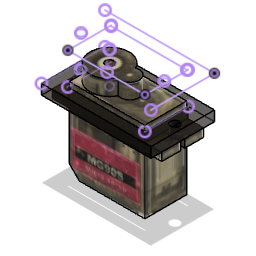
Servo v2 (Autodesk Fusion 360 design; units mm, degrees)
Autodesk Fusion 360 part; units mm, degrees
(part 1 of 2)
sketch "Component_Variables" plane through (0, 0, 0) normal (0, 1, 0) x (1, 0, 0) in component "Servo"
  dimension "tol" = 0
  dimension "tol2" = 0
  dimension "HornScrewtopThickness" = 1.2
  dimension "HornCollarGap" = 0.35
  dimension "HornToServoTopGap" = 0.2
  dimension "HornScrewtopScrewDiaExtra" = 0.4
sketch "Shaft" plane through (0, 0, 0) normal (0, 1, 0) x (1, 0, 0) in component "Shaft"
  circle A0 centre (0, 0) radius 1.25
  circle A1 centre (0, 0) radius 2.4
  circle A2 centre (0, 0) radius 2.25 construction
  line L0 (0, 0) -> (0, 2.4) construction
  line L1 (0, 0) -> (-0.741641, 2.282536) construction
  line L2 (-0.695288, 2.139877) -> (0, 2.25) construction
  line L3 (-0.347644, 2.194939) -> (-0.375443, 2.370452) construction
  line L4 (0, 2.4) -> (-4, 2.4) construction
  line L5 (-0.351978, 2.222299) -> (-1.537204, 2.034577) construction
  spline S0 degree 5 poles (0, 2.4) (-0.019472, 2.4) (-0.055772, 2.396788) (-0.102302, 2.382342) (-0.151568, 2.347419) (-0.205208, 2.293022) (-0.253386, 2.253987) (-0.298375, 2.233713) (-0.333289, 2.225259) (-0.351978, 2.222299) knots 0 0 0 0 0 0 0.2 0.4 0.6 0.8 1 1 1 1 1 1
  line L6 (0.047124, 2.4) -> (-0.047124, 2.4)
  line L7 (-0.305434, 2.229671) -> (-0.398521, 2.214927)
  spline S1 degree 5 poles (0, 2.4) (0.019472, 2.4) (0.055772, 2.396788) (0.102302, 2.382342) (0.151568, 2.347419) (0.205208, 2.293022) (0.253386, 2.253987) (0.298375, 2.233713) (0.333289, 2.225259) (0.351978, 2.222299) knots 0 0 0 0 0 0 0.2 0.4 0.6 0.8 1 1 1 1 1 1
  line L8 (-0.047124, 2.4) -> (0.047124, 2.4)
  line L9 (0.305434, 2.229671) -> (0.398521, 2.214927)
  line L10 (0.351978, 2.222299) -> (0, 0)
  line L11 (-0.351978, 2.222299) -> (0, 0)
  circle A3 centre (0, 0) radius 1.75
  spline S2 degree 5 poles (-0.741641, 2.282536) (-0.723122, 2.288553) (-0.687606, 2.296715) (-0.638889, 2.297355) (-0.581243, 2.279365) (-0.513418, 2.244207) (-0.455536, 2.22197) (-0.406484, 2.21659) (-0.370666, 2.219339) (-0.351978, 2.222299) knots 0 0 0 0 0 0 0.2 0.4 0.6 0.8 1 1 1 1 1 1
  line L12 (-0.786458, 2.267974) -> (-0.696823, 2.297098)
  line L13 (-0.398521, 2.214927) -> (-0.305434, 2.229671)
  point P0 (-0.741641, 2.282536)
  point P1 (-1.410685, 1.941641)
  point P2 (-1.941641, 1.410685)
  point P3 (-2.282536, 0.741641)
  point P4 (-0.347644, 2.194939)
  point P5 (-2.4, 0)
  point P6 (-2.282536, -0.741641)
  point P7 (-1.941641, -1.410685)
  point P8 (-1.410685, -1.941641)
  point P9 (-0.741641, -2.282536)
  point P10 (0, -2.4)
  point P11 (0.741641, -2.282536)
  point P12 (1.410685, -1.941641)
  point P13 (1.941641, -1.410685)
  point P14 (2.282536, -0.741641)
  point P15 (2.4, 0)
  point P16 (2.282536, 0.741641)
  point P17 (1.941641, 1.410685)
  point P18 (1.410685, 1.941641)
  point P19 (0.741641, 2.282536)
  dimension "ScrewholeDia" = 2.5
  dimension "ShaftOuterDia" = 4.8
  dimension "ShaftSplinesInnerDia" = 4.5
  dimension "d5" = 360
  dimension "d6" = 4
  dimension "d7" = 1.2
  dimension "SplineTipPointiness" = 0.094248
  dimension "SplineInnerPointiness" = 0.094248
  dimension "d13" = 3.5
  constraint coincident A0.centre A1.centre
  constraint concentric A0 A1
  constraint concentric A0 A2
  constraint coincident A1 L0.end
  constraint vertical L0
  constraint coincident A2 L2.end
  constraint coincident L0 L2.end
  constraint perpendicular L2 L3
  constraint tangent A1 L4
  constraint perpendicular L3 L5
  constraint midpoint L0.end L6
  constraint parallel L4 L6
  constraint parallel L5 L7
  constraint symmetric L4.start L0 S0.start
  constraint concentric A1 A3
  measures "ScrewholeDia" diameter of A0
  measures "ShaftOuterDia" diameter of A1
  measures "ShaftSplinesInnerDia" diameter of A2
  measures "d6" distance of L0.end L4.end
  measures "d13" diameter of A3
extrude "Extrude3" add sketch "Shaft" against normal blind 3.5 contours A0 L10 L11 | A0 L10 L11 A3 | A0 L10 L11 | A0 L10 L11 A3 | S0 S1 L10 L11 A3 | A1 S1 L10 L11 A3 S2 | A1 S0 S2 picked at (0.828843, -0.061007) picked at (1.484688, -0.538585) picked at (-0.086988, 0.827632) picked at (0.143589, 1.574781) picked at (0.030529, 2.097713) picked at (-0.857161, 2.002429) picked at (-0.367278, 2.318902) makes body 1 in component "Shaft"
extrude "Extrude4" cut sketch "Shaft" against normal blind 3.5 contours A0 L10 L11 | A0 L10 L11 | A1 S0 S2 picked at (0.828843, -0.061007) picked at (-0.086988, 0.827632) picked at (-0.367278, 2.318902) bodies 1 in component "Shaft"
pattern_circular "C-Pattern3" count 20 over 360 about axis through (0, 1.75, 0) along (0, 1, 0) of "Extrude4" in component "Shaft"
extrude "Ignore" add sketch "Shaft" along normal blind 3.5 separate body contours A0 L10 L11 A3 | S0 S1 L10 L11 A3 picked at (-0.186964, 1.570222) picked at (-0.030529, 2.097713) makes body 2 in component "Shaft"
coil "CoilPrimitive1" add diameter 2.5 section triangle in size 0.2 inside turns 8.75 pitch 0.4 right hand placed x (1, 0, 0) y (0, 0, 1) z (0, -1, 0) at (0, 0, 0) separate body makes body 3 in component "Shaft"
extrude "Extrude5" add sketch "Shaft" against normal blind 3.5 separate body contours A0 L10 L11 | A0 L10 L11 picked at (0.828843, -0.061007) picked at (0.086988, 0.827632) makes body 4 in component "Shaft"
combine "Combine2" operation intersect target body 4 tool bodies 3 in component "Shaft"
sketch "Hat" plane through (0, -3.5, 0) normal (0, -1, 0) x (1, 0, 0) in component "Servo"
  circle A0 centre (0, 0) radius 1.25
  spline S0 degree 5 poles (0, -2.4) (0.019472, -2.4) (0.055772, -2.396788) (0.102302, -2.382342) (0.151568, -2.347419) (0.205208, -2.293022) (0.253386, -2.253987) (0.298375, -2.233713) (0.333289, -2.225259) (0.351978, -2.222299) knots 0 0 0 0 0 0 0.2 0.4 0.6 0.8 1 1 1 1 1 1
  spline S1 degree 5 poles (0.351978, -2.222299) (0.370666, -2.219339) (0.406484, -2.21659) (0.455536, -2.22197) (0.513418, -2.244207) (0.581243, -2.279365) (0.638889, -2.297355) (0.687606, -2.296715) (0.723122, -2.288553) (0.741641, -2.282536) knots -1 -1 -1 -1 -1 -1 -0.8 -0.6 -0.4 -0.2 0 0 0 0 0 0
  spline S2 degree 5 poles (0.741641, -2.282536) (0.760159, -2.276519) (0.79369, -2.262246) (0.833479, -2.234128) (0.869542, -2.185691) (0.903747, -2.117381) (0.937505, -2.065369) (0.974026, -2.032184) (1.004619, -2.013355) (1.021479, -2.004765) knots 0 0 0 0 0 0 0.2 0.4 0.6 0.8 1 1 1 1 1 1
  spline S3 degree 5 poles (1.021479, -2.004765) (1.038338, -1.996174) (1.071553, -1.982492) (1.119867, -1.972451) (1.181788, -1.975712) (1.257157, -1.988191) (1.317541, -1.987487) (1.363676, -1.971824) (1.394932, -1.953086) (1.410685, -1.941641) knots -1 -1 -1 -1 -1 -1 -0.8 -0.6 -0.4 -0.2 0 0 0 0 0 0
  spline S4 degree 5 poles (1.410685, -1.941641) (1.426437, -1.930196) (1.453917, -1.90626) (1.483069, -1.867223) (1.502399, -1.810012) (1.513821, -1.734476) (1.529854, -1.674577) (1.554334, -1.631731) (1.577611, -1.60437) (1.59099, -1.59099) knots 0 0 0 0 0 0 0.2 0.4 0.6 0.8 1 1 1 1 1 1
  spline S5 degree 5 poles (1.59099, -1.59099) (1.60437, -1.577611) (1.631731, -1.554334) (1.674577, -1.529854) (1.734476, -1.513821) (1.810012, -1.502399) (1.867223, -1.483069) (1.90626, -1.453917) (1.930196, -1.426437) (1.941641, -1.410685) knots -1 -1 -1 -1 -1 -1 -0.8 -0.6 -0.4 -0.2 0 0 0 0 0 0
  spline S6 degree 5 poles (1.941641, -1.410685) (1.953086, -1.394932) (1.971824, -1.363676) (1.987487, -1.317541) (1.988191, -1.257157) (1.975712, -1.181788) (1.972451, -1.119867) (1.982492, -1.071553) (1.996174, -1.038338) (2.004765, -1.021479) knots 0 0 0 0 0 0 0.2 0.4 0.6 0.8 1 1 1 1 1 1
  spline S7 degree 5 poles (2.004765, -1.021479) (2.013355, -1.004619) (2.032184, -0.974026) (2.065369, -0.937505) (2.117381, -0.903747) (2.185691, -0.869542) (2.234128, -0.833479) (2.262246, -0.79369) (2.276519, -0.760159) (2.282536, -0.741641) knots -1 -1 -1 -1 -1 -1 -0.8 -0.6 -0.4 -0.2 0 0 0 0 0 0
  spline S8 degree 5 poles (2.282536, -0.741641) (2.288553, -0.723122) (2.296715, -0.687606) (2.297355, -0.638889) (2.279365, -0.581243) (2.244207, -0.513418) (2.22197, -0.455536) (2.21659, -0.406484) (2.219339, -0.370666) (2.222299, -0.351978) knots 0 0 0 0 0 0 0.2 0.4 0.6 0.8 1 1 1 1 1 1
  spline S9 degree 5 poles (2.222299, -0.351978) (2.225259, -0.333289) (2.233713, -0.298375) (2.253987, -0.253386) (2.293022, -0.205208) (2.347419, -0.151568) (2.382342, -0.102302) (2.396788, -0.055772) (2.4, -0.019472) (2.4, 0) knots -1 -1 -1 -1 -1 -1 -0.8 -0.6 -0.4 -0.2 0 0 0 0 0 0
  spline S10 degree 5 poles (2.4, 0) (2.4, 0.019472) (2.396788, 0.055772) (2.382342, 0.102302) (2.347419, 0.151568) (2.293022, 0.205208) (2.253987, 0.253386) (2.233713, 0.298375) (2.225259, 0.333289) (2.222299, 0.351978) knots 0 0 0 0 0 0 0.2 0.4 0.6 0.8 1 1 1 1 1 1
  spline S11 degree 5 poles (2.222299, 0.351978) (2.219339, 0.370666) (2.21659, 0.406484) (2.22197, 0.455536) (2.244207, 0.513418) (2.279365, 0.581243) (2.297355, 0.638889) (2.296715, 0.687606) (2.288553, 0.723122) (2.282536, 0.741641) knots -1 -1 -1 -1 -1 -1 -0.8 -0.6 -0.4 -0.2 0 0 0 0 0 0
  spline S12 degree 5 poles (2.282536, 0.741641) (2.276519, 0.760159) (2.262246, 0.79369) (2.234128, 0.833479) (2.185691, 0.869542) (2.117381, 0.903747) (2.065369, 0.937505) (2.032184, 0.974026) (2.013355, 1.004619) (2.004765, 1.021479) knots 0 0 0 0 0 0 0.2 0.4 0.6 0.8 1 1 1 1 1 1
  spline S13 degree 5 poles (2.004765, 1.021479) (1.996174, 1.038338) (1.982492, 1.071553) (1.972451, 1.119867) (1.975712, 1.181788) (1.988191, 1.257157) (1.987487, 1.317541) (1.971824, 1.363676) (1.953086, 1.394932) (1.941641, 1.410685) knots -1 -1 -1 -1 -1 -1 -0.8 -0.6 -0.4 -0.2 0 0 0 0 0 0
  spline S14 degree 5 poles (1.941641, 1.410685) (1.930196, 1.426437) (1.90626, 1.453917) (1.867223, 1.483069) (1.810012, 1.502399) (1.734476, 1.513821) (1.674577, 1.529854) (1.631731, 1.554334) (1.60437, 1.577611) (1.59099, 1.59099) knots 0 0 0 0 0 0 0.2 0.4 0.6 0.8 1 1 1 1 1 1
  spline S15 degree 5 poles (1.59099, 1.59099) (1.577611, 1.60437) (1.554334, 1.631731) (1.529854, 1.674577) (1.513821, 1.734476) (1.502399, 1.810012) (1.483069, 1.867223) (1.453917, 1.90626) (1.426437, 1.930196) (1.410685, 1.941641) knots -1 -1 -1 -1 -1 -1 -0.8 -0.6 -0.4 -0.2 0 0 0 0 0 0
  spline S16 degree 5 poles (1.410685, 1.941641) (1.394932, 1.953086) (1.363676, 1.971824) (1.317541, 1.987487) (1.257157, 1.988191) (1.181788, 1.975712) (1.119867, 1.972451) (1.071553, 1.982492) (1.038338, 1.996174) (1.021479, 2.004765) knots 0 0 0 0 0 0 0.2 0.4 0.6 0.8 1 1 1 1 1 1
  spline S17 degree 5 poles (1.021479, 2.004765) (1.004619, 2.013355) (0.974026, 2.032184) (0.937505, 2.065369) (0.903747, 2.117381) (0.869542, 2.185691) (0.833479, 2.234128) (0.79369, 2.262246) (0.760159, 2.276519) (0.741641, 2.282536) knots -1 -1 -1 -1 -1 -1 -0.8 -0.6 -0.4 -0.2 0 0 0 0 0 0
  spline S18 degree 5 poles (0.741641, 2.282536) (0.723122, 2.288553) (0.687606, 2.296715) (0.638889, 2.297355) (0.581243, 2.279365) (0.513418, 2.244207) (0.455536, 2.22197) (0.406484, 2.21659) (0.370666, 2.219339) (0.351978, 2.222299) knots 0 0 0 0 0 0 0.2 0.4 0.6 0.8 1 1 1 1 1 1
  spline S19 degree 5 poles (0.351978, 2.222299) (0.333289, 2.225259) (0.298375, 2.233713) (0.253386, 2.253987) (0.205208, 2.293022) (0.151568, 2.347419) (0.102302, 2.382342) (0.055772, 2.396788) (0.019472, 2.4) (0, 2.4) knots -1 -1 -1 -1 -1 -1 -0.8 -0.6 -0.4 -0.2 0 0 0 0 0 0
  spline S20 degree 5 poles (0, 2.4) (-0.019472, 2.4) (-0.055772, 2.396788) (-0.102302, 2.382342) (-0.151568, 2.347419) (-0.205208, 2.293022) (-0.253386, 2.253987) (-0.298375, 2.233713) (-0.333289, 2.225259) (-0.351978, 2.222299) knots 0 0 0 0 0 0 0.2 0.4 0.6 0.8 1 1 1 1 1 1
  spline S21 degree 5 poles (-0.351978, 2.222299) (-0.370666, 2.219339) (-0.406484, 2.21659) (-0.455536, 2.22197) (-0.513418, 2.244207) (-0.581243, 2.279365) (-0.638889, 2.297355) (-0.687606, 2.296715) (-0.723122, 2.288553) (-0.741641, 2.282536) knots -1 -1 -1 -1 -1 -1 -0.8 -0.6 -0.4 -0.2 0 0 0 0 0 0
  spline S22 degree 5 poles (-0.741641, 2.282536) (-0.760159, 2.276519) (-0.79369, 2.262246) (-0.833479, 2.234128) (-0.869542, 2.185691) (-0.903747, 2.117381) (-0.937505, 2.065369) (-0.974026, 2.032184) (-1.004619, 2.013355) (-1.021479, 2.004765) knots 0 0 0 0 0 0 0.2 0.4 0.6 0.8 1 1 1 1 1 1
  spline S23 degree 5 poles (-1.021479, 2.004765) (-1.038338, 1.996174) (-1.071553, 1.982492) (-1.119867, 1.972451) (-1.181788, 1.975712) (-1.257157, 1.988191) (-1.317541, 1.987487) (-1.363676, 1.971824) (-1.394932, 1.953086) (-1.410685, 1.941641) knots -1 -1 -1 -1 -1 -1 -0.8 -0.6 -0.4 -0.2 0 0 0 0 0 0
  spline S24 degree 5 poles (-1.410685, 1.941641) (-1.426437, 1.930196) (-1.453917, 1.90626) (-1.483069, 1.867223) (-1.502399, 1.810012) (-1.513821, 1.734476) (-1.529854, 1.674577) (-1.554334, 1.631731) (-1.577611, 1.60437) (-1.59099, 1.59099) knots 0 0 0 0 0 0 0.2 0.4 0.6 0.8 1 1 1 1 1 1
  spline S25 degree 5 poles (-1.59099, 1.59099) (-1.60437, 1.577611) (-1.631731, 1.554334) (-1.674577, 1.529854) (-1.734476, 1.513821) (-1.810012, 1.502399) (-1.867223, 1.483069) (-1.90626, 1.453917) (-1.930196, 1.426437) (-1.941641, 1.410685) knots -1 -1 -1 -1 -1 -1 -0.8 -0.6 -0.4 -0.2 0 0 0 0 0 0
  spline S26 degree 5 poles (-1.941641, 1.410685) (-1.953086, 1.394932) (-1.971824, 1.363676) (-1.987487, 1.317541) (-1.988191, 1.257157) (-1.975712, 1.181788) (-1.972451, 1.119867) (-1.982492, 1.071553) (-1.996174, 1.038338) (-2.004765, 1.021479) knots 0 0 0 0 0 0 0.2 0.4 0.6 0.8 1 1 1 1 1 1
  spline S27 degree 5 poles (-2.004765, 1.021479) (-2.013355, 1.004619) (-2.032184, 0.974026) (-2.065369, 0.937505) (-2.117381, 0.903747) (-2.185691, 0.869542) (-2.234128, 0.833479) (-2.262246, 0.79369) (-2.276519, 0.760159) (-2.282536, 0.741641) knots -1 -1 -1 -1 -1 -1 -0.8 -0.6 -0.4 -0.2 0 0 0 0 0 0
  spline S28 degree 5 poles (-2.282536, 0.741641) (-2.288553, 0.723122) (-2.296715, 0.687606) (-2.297355, 0.638889) (-2.279365, 0.581243) (-2.244207, 0.513418) (-2.22197, 0.455536) (-2.21659, 0.406484) (-2.219339, 0.370666) (-2.222299, 0.351978) knots 0 0 0 0 0 0 0.2 0.4 0.6 0.8 1 1 1 1 1 1
  spline S29 degree 5 poles (-2.222299, 0.351978) (-2.225259, 0.333289) (-2.233713, 0.298375) (-2.253987, 0.253386) (-2.293022, 0.205208) (-2.347419, 0.151568) (-2.382342, 0.102302) (-2.396788, 0.055772) (-2.4, 0.019472) (-2.4, 0) knots -1 -1 -1 -1 -1 -1 -0.8 -0.6 -0.4 -0.2 0 0 0 0 0 0
  spline S30 degree 5 poles (-2.4, 0) (-2.4, -0.019472) (-2.396788, -0.055772) (-2.382342, -0.102302) (-2.347419, -0.151568) (-2.293022, -0.205208) (-2.253987, -0.253386) (-2.233713, -0.298375) (-2.225259, -0.333289) (-2.222299, -0.351978) knots 0 0 0 0 0 0 0.2 0.4 0.6 0.8 1 1 1 1 1 1
  spline S31 degree 5 poles (-2.222299, -0.351978) (-2.219339, -0.370666) (-2.21659, -0.406484) (-2.22197, -0.455536) (-2.244207, -0.513418) (-2.279365, -0.581243) (-2.297355, -0.638889) (-2.296715, -0.687606) (-2.288553, -0.723122) (-2.282536, -0.741641) knots -1 -1 -1 -1 -1 -1 -0.8 -0.6 -0.4 -0.2 0 0 0 0 0 0
  spline S32 degree 5 poles (-2.282536, -0.741641) (-2.276519, -0.760159) (-2.262246, -0.79369) (-2.234128, -0.833479) (-2.185691, -0.869542) (-2.117381, -0.903747) (-2.065369, -0.937505) (-2.032184, -0.974026) (-2.013355, -1.004619) (-2.004765, -1.021479) knots 0 0 0 0 0 0 0.2 0.4 0.6 0.8 1 1 1 1 1 1
  spline S33 degree 5 poles (-2.004765, -1.021479) (-1.996174, -1.038338) (-1.982492, -1.071553) (-1.972451, -1.119867) (-1.975712, -1.181788) (-1.988191, -1.257157) (-1.987487, -1.317541) (-1.971824, -1.363676) (-1.953086, -1.394932) (-1.941641, -1.410685) knots -1 -1 -1 -1 -1 -1 -0.8 -0.6 -0.4 -0.2 0 0 0 0 0 0
  spline S34 degree 5 poles (-1.941641, -1.410685) (-1.930196, -1.426437) (-1.90626, -1.453917) (-1.867223, -1.483069) (-1.810012, -1.502399) (-1.734476, -1.513821) (-1.674577, -1.529854) (-1.631731, -1.554334) (-1.60437, -1.577611) (-1.59099, -1.59099) knots 0 0 0 0 0 0 0.2 0.4 0.6 0.8 1 1 1 1 1 1
  spline S35 degree 5 poles (-1.59099, -1.59099) (-1.577611, -1.60437) (-1.554334, -1.631731) (-1.529854, -1.674577) (-1.513821, -1.734476) (-1.502399, -1.810012) (-1.483069, -1.867223) (-1.453917, -1.90626) (-1.426437, -1.930196) (-1.410685, -1.941641) knots -1 -1 -1 -1 -1 -1 -0.8 -0.6 -0.4 -0.2 0 0 0 0 0 0
  spline S36 degree 5 poles (-1.410685, -1.941641) (-1.394932, -1.953086) (-1.363676, -1.971824) (-1.317541, -1.987487) (-1.257157, -1.988191) (-1.181788, -1.975712) (-1.119867, -1.972451) (-1.071553, -1.982492) (-1.038338, -1.996174) (-1.021479, -2.004765) knots 0 0 0 0 0 0 0.2 0.4 0.6 0.8 1 1 1 1 1 1
  spline S37 degree 5 poles (-1.021479, -2.004765) (-1.004619, -2.013355) (-0.974026, -2.032184) (-0.937505, -2.065369) (-0.903747, -2.117381) (-0.869542, -2.185691) (-0.833479, -2.234128) (-0.79369, -2.262246) (-0.760159, -2.276519) (-0.741641, -2.282536) knots -1 -1 -1 -1 -1 -1 -0.8 -0.6 -0.4 -0.2 0 0 0 0 0 0
  spline S38 degree 5 poles (-0.741641, -2.282536) (-0.723122, -2.288553) (-0.687606, -2.296715) (-0.638889, -2.297355) (-0.581243, -2.279365) (-0.513418, -2.244207) (-0.455536, -2.22197) (-0.406484, -2.21659) (-0.370666, -2.219339) (-0.351978, -2.222299) knots 0 0 0 0 0 0 0.2 0.4 0.6 0.8 1 1 1 1 1 1
  spline S39 degree 5 poles (-0.351978, -2.222299) (-0.333289, -2.225259) (-0.298375, -2.233713) (-0.253386, -2.253987) (-0.205208, -2.293022) (-0.151568, -2.347419) (-0.102302, -2.382342) (-0.055772, -2.396788) (-0.019472, -2.4) (0, -2.4) knots -1 -1 -1 -1 -1 -1 -0.8 -0.6 -0.4 -0.2 0 0 0 0 0 0
  circle A1 centre (0, 0) radius 5.75
  line L0 (0, 0) -> (-5.75, 0) construction
  line L1 (-5.75, 0) -> (8.75, 0) construction
  circle A2 centre (6, 0) radius 2.75
  line L2 (8.75, 0) -> (6, 0) construction
  dimension "HatDia" = 11.5
  dimension "HatLen" = 14.5
  dimension "HatTipDia" = 5.5
  dimension "d36" = 2.75
  constraint concentric A0 A1
  constraint coincident A0.centre A1.centre
  constraint coincident A1 L0.end
  constraint horizontal L0
  constraint parallel L0 L1
  constraint parallel L1 L2
  constraint coincident A2.centre L2.end
  measures "HatDia" diameter of A1
  measures "HatLen" distance of L0.end L1.end
  measures "HatTipDia" diameter of A2
  measures "d36" distance of L1.end A2.centre
extrude "Extrude1" add sketch "Hat" along normal blind 4.5 separate body contours S0 S1 S2 S3 S4 S5 S6 S7 S8 S9 S10 S11 S12 S13 S14 S15 S16 S17 S18 S19 S20 S21 S22 S23 S24 S25 S26 S27 S28 S29 S30 S31 S32 S33 S34 S35 S36 S37 S38 S39 | A1 A2 | A1 A2 | A1 A2 picked at (-1.922941, 0.00022) picked at (4.925523, -0.425062) picked at (6.698087, 0.488389) picked at (3.22932, 2.627359) makes body 5 in component "Servo"
sketch "ServoBody" plane through (0, -8, 0) normal (0, -1, 0) x (1, 0, 0) in component "Servo"
  circle A0 centre (0, 0) radius 1.25
  arc A1 (5.125, -2.607082) -> (5.125, 2.607082) centre (6, 0) ccw
  arc A2 (5.125, 2.607082) -> (5.125, -2.607082) centre (0, 0) ccw
  line L0 (0, 0) -> (-5.75, 0) construction
  line L1 (-5.75, 0) -> (16.65, 0) construction
  line L2 (16.65, 0) -> (16.65, 12.4)
  line L3 (16.65, 6.2) -> (-5.75, 6.2)
  line L4 (-5.75, 6.2) -> (-5.75, 0)
  line L5 (16.65, 0) -> (16.65, -12.4)
  line L6 (16.65, -6.2) -> (-5.75, -6.2)
  line L7 (-5.75, -6.2) -> (-5.75, 0)
  dimension "Hole_to_closest_end_dist" = 5.75
  dimension "ServoBodyLength" = 22.4
  dimension "ServoBodyWidth" = 12.4
  constraint coincident A0.centre A2.centre
  constraint horizontal L0
  constraint parallel L0 L1
  constraint perpendicular L1 L2
  constraint midpoint L2 L3.start
  constraint perpendicular L2 L3
  constraint perpendicular L1 L4
  constraint symmetric L0.end L1 L4.end
  constraint symmetric L2.start L1 L5.start
  constraint symmetric L1 L2.end L5.end
  constraint symmetric L1 L3.start L6.start
  constraint symmetric L1 L3.end L6.end
  measures "Hole_to_closest_end_dist" distance of A0.centre L0.end
  measures "ServoBodyLength" distance of L0.end L1.end
  measures "ServoBodyWidth" distance of L1.end L2.end
extrude "Extrude2" add sketch "ServoBody" along normal blind 24 contours A1 A2 | L2 L3 L4 L5 L6 L7 picked at (3.833333, 0) picked at (13.930439, -2.454802) bodies 5 in component "Servo"
chamfer "Chamfer1" distance 3 angle 45 1 edges at (-5.75, -32, 0) on bodies 5 in component "Servo"
ref_plane "WorkPlane1" through (5.45, -12.4, 0) normal (0, 1, 0) x (-1, 0, 0) in component "Servo"
sketch "ScrewTab" plane through (5.45, -12.4, 0) normal (0, 1, 0) x (1, 0, 0) in component "Servo"
  line L0 (11.2, -6.2) -> (-11.2, -6.2)
  line L1 (-11.2, -6.2) -> (-11.2, 0)
  line L2 (-11.2, 6.2) -> (-11.2, 0)
  line L3 (11.2, 6.2) -> (-11.2, 6.2)
  line L4 (11.2, 0) -> (11.2, 12.4)
  line L5 (11.2, 0) -> (11.2, -12.4)
  line L6 (-11.2, 0) -> (11.2, 0)
  line L7 (-11.2, -6.2) -> (-16.2, -6.2)
  line L8 (-16.2, -6.2) -> (-16.2, 6.2) construction
  line L9 (-16.2, 6.2) -> (-11.2, 6.2)
  line L10 (-11.2, 6.2) -> (-11.2, -6.2)
  line L11 (11.2, -6.2) -> (16.2, -6.2)
  line L12 (16.2, -6.2) -> (16.2, 6.2) construction
  line L13 (16.2, 6.2) -> (11.2, 6.2)
  line L14 (11.2, 6.2) -> (11.2, -6.2)
  line L15 (16.2, 0) -> (12.6, 0) construction
  circle A0 centre (13.9, 0) radius 1.3
  line L16 (12.6, 0) -> (13.9, 0) construction
  line L17 (16.2, 0) -> (-16.2, 0) construction
  line L18 (0, 0) -> (0, -6.2) construction
  line L19 (13.9, 0) -> (13.9, -1.2) construction
  line L20 (16.2, -6.2) -> (16.2, -0.6)
  line L21 (16.2, -0.6) -> (15.053256, -0.6)
  line L22 (16.2, 0.6) -> (15.053256, 0.6)
  line L23 (16.2, 6.2) -> (16.2, 0.6)
  circle A1 centre (-13.9, 0) radius 1.3
  line L24 (-16.2, 0.6) -> (-15.053256, 0.6)
  line L25 (-16.2, -0.6) -> (-15.053256, -0.6)
  line L26 (-16.2, -6.2) -> (-16.2, -0.6)
  line L27 (-16.2, 6.2) -> (-16.2, 0.6)
  dimension "ServoTabSize" = 5
  dimension "d47" = 12.4
  dimension "d48" = 5
  dimension "d49" = 12.4
  dimension "ServoHoleRecess" = 3.6
  dimension "TabScrewSize" = 2.6
  dimension "d52" = 1.3
  dimension "d53" = 6.2
  dimension "TabScrewGapSize" = 1.2
  dimension "d55" = 5.6
  constraint horizontal L7
  constraint vertical L8
  constraint horizontal L9
  constraint vertical L10
  constraint coincident L0.end L1.start
  constraint horizontal L11
  constraint vertical L12
  constraint horizontal L13
  constraint vertical L14
  constraint coincident L0.start L11.start
  constraint midpoint L12 L15.start
  constraint perpendicular L12 L15
  constraint perpendicular L12 L16
  constraint coincident A0.centre L16.end
  constraint midpoint L8 L17.end
  constraint coincident L6 L18.start
  constraint perpendicular L6 L18
  constraint midpoint L17 L18.start
  constraint perpendicular L17 L19
  constraint perpendicular L11 L20
  constraint perpendicular L20 L21
  constraint symmetric L11.end L15 L12.end
  constraint symmetric L15 L20.end L22.start
  constraint symmetric L11.end L18 L7.end
  constraint symmetric A0 L18 A1
  constraint symmetric L18 L20.end L25.start
  constraint symmetric L18 L22.start L24.start
  constraint symmetric L18 L12.end L8.end
  measures "ServoTabSize" distance of L0.end L7.end
  measures "d47" distance of L0.end L2.start
  measures "d48" distance of L0.start L11.end
  measures "d49" distance of L0.start L3.start
  measures "ServoHoleRecess" distance of L15.start L15.end
  measures "TabScrewSize" diameter of A0
  measures "d52" distance of L15.end A0.centre
  measures "d53" distance of L18.start L18.end
  measures "TabScrewGapSize" distance of A0.centre L19.end
  measures "d55" distance of L11.end L20.end
extrude "Extrude3'" add sketch "ScrewTab" against normal blind 2.4 contours L4 L5 L11 L13 L14 A0 L20 L21 L22 L23 | L1 L2 L7 L9 L10 A1 L24 L25 L26 L27 picked at (13.726864, -4.564835) picked at (-13.726864, 4.564835) bodies 5 in component "Servo"
sketch "WireHole" plane through (-17.375, -17.375, 0) normal (-0.70710678, -0.70710678, 0) x (0, 0, 1) in component "Servo"
  line L0 (-6.2, -16.440233) -> (-6.2, -20.682873) construction
  line L1 (-6.2, -20.682873) -> (6.2, -20.682873) construction
  line L2 (6.2, -20.682873) -> (6.2, -16.440233) construction
  line L3 (6.2, -16.440233) -> (-6.2, -16.440233)
  line L4 (6.2, -16.440233) -> (-6.2, -16.440233) construction
  line L5 (-6.2, -20.682873) -> (6.2, -20.682873) construction
  line L6 (6.2, -20.682873) -> (9.2, -20.682873) construction
  line L7 (9.2, -20.682873) -> (9.2, -20.282873) construction
  line L8 (9.2, -20.282873) -> (9.2, -18.282873) construction
  line L9 (0, -20.282873) -> (0, -18.282873) construction
  line L10 (0, -18.282873) -> (-1.5, -18.282873)
  line L11 (-1.5, -18.282873) -> (1.5, -18.282873)
  line L12 (1.5, -18.282873) -> (1.5, -20.282873)
  line L13 (1.5, -20.282873) -> (-1.5, -20.282873)
  line L14 (-1.5, -20.282873) -> (-1.5, -18.282873)
  line L15 (1.5, -19.282873) -> (-1.5, -19.282873) construction
  circle A0 centre (0, -19.282873) radius 0.375
  line L16 (0, -19.282873) -> (-0.85, -19.282873) construction
  circle A1 centre (-0.85, -19.282873) radius 0.375
  circle A2 centre (0.85, -19.282873) radius 0.375
  dimension "WireHoleWidth" = 3
  dimension "WireHoleOffset" = 0.4
  dimension "WireHoleHeight" = 2
  dimension "d61" = 2
  dimension "d62" = 1.5
  dimension "d63" = 3
  dimension "d64" = 2
  dimension "d65" = 0.75
  dimension "d66" = 0.85
  dimension "d67" = 0.75
  constraint perpendicular L2 L6
  constraint perpendicular L6 L7
  constraint parallel L7 L8
  constraint perpendicular L1 L9
  constraint perpendicular L9 L10
  constraint horizontal L11
  constraint vertical L12
  constraint horizontal L13
  constraint vertical L14
  constraint perpendicular L9 L16
  constraint symmetric L9 A1 A2
  measures "d65" diameter of A0
  measures "d67" diameter of A1
extrude "Extrude4'" cut sketch "WireHole" against normal blind 3 contours L10 L11 L12 L13 L14 picked at (-0.009341, -20.07419) bodies 5 in component "Servo"
extrude "Extrude5'" add sketch "WireHole" along normal blind 5 separate body contours A0 | A1 | A2 picked at (0.091631, -19.124163) picked at (-0.74672, -19.175198) picked at (0.95328, -19.175198) makes body 6 at (-6.187664, -33.276381, -1.202385) makes body 7 at (-5.926527, -33.537518, -0.287267) makes body 8 at (-6.187664, -33.276381, 0.497615) in component "Servo"
sketch "Horn" plane through (0, 0, 0) normal (0, 1, 0) x (1, 0, 0) in component "Horn"
  spline S0 degree 5 poles (0.351978, 2.222299) (0.333289, 2.225259) (0.298375, 2.233713) (0.253386, 2.253987) (0.205208, 2.293022) (0.151568, 2.347419) (0.102302, 2.382342) (0.055772, 2.396788) (0.019472, 2.4) (0, 2.4) knots -1 -1 -1 -1 -1 -1 -0.8 -0.6 -0.4 -0.2 0 0 0 0 0 0
  spline S1 degree 5 poles (0, 2.4) (-0.019472, 2.4) (-0.055772, 2.396788) (-0.102302, 2.382342) (-0.151568, 2.347419) (-0.205208, 2.293022) (-0.253386, 2.253987) (-0.298375, 2.233713) (-0.333289, 2.225259) (-0.351978, 2.222299) knots 0 0 0 0 0 0 0.2 0.4 0.6 0.8 1 1 1 1 1 1
  spline S2 degree 5 poles (-0.351978, 2.222299) (-0.370666, 2.219339) (-0.406484, 2.21659) (-0.455536, 2.22197) (-0.513418, 2.244207) (-0.581243, 2.279365) (-0.638889, 2.297355) (-0.687606, 2.296715) (-0.723122, 2.288553) (-0.741641, 2.282536) knots -1 -1 -1 -1 -1 -1 -0.8 -0.6 -0.4 -0.2 0 0 0 0 0 0
  spline S3 degree 5 poles (-0.741641, 2.282536) (-0.760159, 2.276519) (-0.79369, 2.262246) (-0.833479, 2.234128) (-0.869542, 2.185691) (-0.903747, 2.117381) (-0.937505, 2.065369) (-0.974026, 2.032184) (-1.004619, 2.013355) (-1.021479, 2.004765) knots 0 0 0 0 0 0 0.2 0.4 0.6 0.8 1 1 1 1 1 1
  spline S4 degree 5 poles (-1.021479, 2.004765) (-1.038338, 1.996174) (-1.071553, 1.982492) (-1.119867, 1.972451) (-1.181788, 1.975712) (-1.257157, 1.988191) (-1.317541, 1.987487) (-1.363676, 1.971824) (-1.394932, 1.953086) (-1.410685, 1.941641) knots -1 -1 -1 -1 -1 -1 -0.8 -0.6 -0.4 -0.2 0 0 0 0 0 0
  spline S5 degree 5 poles (-1.410685, 1.941641) (-1.426437, 1.930196) (-1.453917, 1.90626) (-1.483069, 1.867223) (-1.502399, 1.810012) (-1.513821, 1.734476) (-1.529854, 1.674577) (-1.554334, 1.631731) (-1.577611, 1.60437) (-1.59099, 1.59099) knots 0 0 0 0 0 0 0.2 0.4 0.6 0.8 1 1 1 1 1 1
  spline S6 degree 5 poles (-1.59099, 1.59099) (-1.60437, 1.577611) (-1.631731, 1.554334) (-1.674577, 1.529854) (-1.734476, 1.513821) (-1.810012, 1.502399) (-1.867223, 1.483069) (-1.90626, 1.453917) (-1.930196, 1.426437) (-1.941641, 1.410685) knots -1 -1 -1 -1 -1 -1 -0.8 -0.6 -0.4 -0.2 0 0 0 0 0 0
  spline S7 degree 5 poles (-1.941641, 1.410685) (-1.953086, 1.394932) (-1.971824, 1.363676) (-1.987487, 1.317541) (-1.988191, 1.257157) (-1.975712, 1.181788) (-1.972451, 1.119867) (-1.982492, 1.071553) (-1.996174, 1.038338) (-2.004765, 1.021479) knots 0 0 0 0 0 0 0.2 0.4 0.6 0.8 1 1 1 1 1 1
  spline S8 degree 5 poles (-2.004765, 1.021479) (-2.013355, 1.004619) (-2.032184, 0.974026) (-2.065369, 0.937505) (-2.117381, 0.903747) (-2.185691, 0.869542) (-2.234128, 0.833479) (-2.262246, 0.79369) (-2.276519, 0.760159) (-2.282536, 0.741641) knots -1 -1 -1 -1 -1 -1 -0.8 -0.6 -0.4 -0.2 0 0 0 0 0 0
  spline S9 degree 5 poles (-2.282536, 0.741641) (-2.288553, 0.723122) (-2.296715, 0.687606) (-2.297355, 0.638889) (-2.279365, 0.581243) (-2.244207, 0.513418) (-2.22197, 0.455536) (-2.21659, 0.406484) (-2.219339, 0.370666) (-2.222299, 0.351978) knots 0 0 0 0 0 0 0.2 0.4 0.6 0.8 1 1 1 1 1 1
  spline S10 degree 5 poles (-2.222299, 0.351978) (-2.225259, 0.333289) (-2.233713, 0.298375) (-2.253987, 0.253386) (-2.293022, 0.205208) (-2.347419, 0.151568) (-2.382342, 0.102302) (-2.396788, 0.055772) (-2.4, 0.019472) (-2.4, 0) knots -1 -1 -1 -1 -1 -1 -0.8 -0.6 -0.4 -0.2 0 0 0 0 0 0
  spline S11 degree 5 poles (-2.4, 0) (-2.4, -0.019472) (-2.396788, -0.055772) (-2.382342, -0.102302) (-2.347419, -0.151568) (-2.293022, -0.205208) (-2.253987, -0.253386) (-2.233713, -0.298375) (-2.225259, -0.333289) (-2.222299, -0.351978) knots 0 0 0 0 0 0 0.2 0.4 0.6 0.8 1 1 1 1 1 1
  spline S12 degree 5 poles (-2.222299, -0.351978) (-2.219339, -0.370666) (-2.21659, -0.406484) (-2.22197, -0.455536) (-2.244207, -0.513418) (-2.279365, -0.581243) (-2.297355, -0.638889) (-2.296715, -0.687606) (-2.288553, -0.723122) (-2.282536, -0.741641) knots -1 -1 -1 -1 -1 -1 -0.8 -0.6 -0.4 -0.2 0 0 0 0 0 0
  spline S13 degree 5 poles (-2.282536, -0.741641) (-2.276519, -0.760159) (-2.262246, -0.79369) (-2.234128, -0.833479) (-2.185691, -0.869542) (-2.117381, -0.903747) (-2.065369, -0.937505) (-2.032184, -0.974026) (-2.013355, -1.004619) (-2.004765, -1.021479) knots 0 0 0 0 0 0 0.2 0.4 0.6 0.8 1 1 1 1 1 1
  spline S14 degree 5 poles (-2.004765, -1.021479) (-1.996174, -1.038338) (-1.982492, -1.071553) (-1.972451, -1.119867) (-1.975712, -1.181788) (-1.988191, -1.257157) (-1.987487, -1.317541) (-1.971824, -1.363676) (-1.953086, -1.394932) (-1.941641, -1.410685) knots -1 -1 -1 -1 -1 -1 -0.8 -0.6 -0.4 -0.2 0 0 0 0 0 0
  spline S15 degree 5 poles (-1.941641, -1.410685) (-1.930196, -1.426437) (-1.90626, -1.453917) (-1.867223, -1.483069) (-1.810012, -1.502399) (-1.734476, -1.513821) (-1.674577, -1.529854) (-1.631731, -1.554334) (-1.60437, -1.577611) (-1.59099, -1.59099) knots 0 0 0 0 0 0 0.2 0.4 0.6 0.8 1 1 1 1 1 1
  spline S16 degree 5 poles (-1.59099, -1.59099) (-1.577611, -1.60437) (-1.554334, -1.631731) (-1.529854, -1.674577) (-1.513821, -1.734476) (-1.502399, -1.810012) (-1.483069, -1.867223) (-1.453917, -1.90626) (-1.426437, -1.930196) (-1.410685, -1.941641) knots -1 -1 -1 -1 -1 -1 -0.8 -0.6 -0.4 -0.2 0 0 0 0 0 0
  spline S17 degree 5 poles (-1.410685, -1.941641) (-1.394932, -1.953086) (-1.363676, -1.971824) (-1.317541, -1.987487) (-1.257157, -1.988191) (-1.181788, -1.975712) (-1.119867, -1.972451) (-1.071553, -1.982492) (-1.038338, -1.996174) (-1.021479, -2.004765) knots 0 0 0 0 0 0 0.2 0.4 0.6 0.8 1 1 1 1 1 1
  spline S18 degree 5 poles (-1.021479, -2.004765) (-1.004619, -2.013355) (-0.974026, -2.032184) (-0.937505, -2.065369) (-0.903747, -2.117381) (-0.869542, -2.185691) (-0.833479, -2.234128) (-0.79369, -2.262246) (-0.760159, -2.276519) (-0.741641, -2.282536) knots -1 -1 -1 -1 -1 -1 -0.8 -0.6 -0.4 -0.2 0 0 0 0 0 0
  spline S19 degree 5 poles (-0.741641, -2.282536) (-0.723122, -2.288553) (-0.687606, -2.296715) (-0.638889, -2.297355) (-0.581243, -2.279365) (-0.513418, -2.244207) (-0.455536, -2.22197) (-0.406484, -2.21659) (-0.370666, -2.219339) (-0.351978, -2.222299) knots 0 0 0 0 0 0 0.2 0.4 0.6 0.8 1 1 1 1 1 1
  spline S20 degree 5 poles (-0.351978, -2.222299) (-0.333289, -2.225259) (-0.298375, -2.233713) (-0.253386, -2.253987) (-0.205208, -2.293022) (-0.151568, -2.347419) (-0.102302, -2.382342) (-0.055772, -2.396788) (-0.019472, -2.4) (0, -2.4) knots -1 -1 -1 -1 -1 -1 -0.8 -0.6 -0.4 -0.2 0 0 0 0 0 0
  spline S21 degree 5 poles (0, -2.4) (0.019472, -2.4) (0.055772, -2.396788) (0.102302, -2.382342) (0.151568, -2.347419) (0.205208, -2.293022) (0.253386, -2.253987) (0.298375, -2.233713) (0.333289, -2.225259) (0.351978, -2.222299) knots 0 0 0 0 0 0 0.2 0.4 0.6 0.8 1 1 1 1 1 1
  spline S22 degree 5 poles (0.351978, -2.222299) (0.370666, -2.219339) (0.406484, -2.21659) (0.455536, -2.22197) (0.513418, -2.244207) (0.581243, -2.279365) (0.638889, -2.297355) (0.687606, -2.296715) (0.723122, -2.288553) (0.741641, -2.282536) knots -1 -1 -1 -1 -1 -1 -0.8 -0.6 -0.4 -0.2 0 0 0 0 0 0
  spline S23 degree 5 poles (0.741641, -2.282536) (0.760159, -2.276519) (0.79369, -2.262246) (0.833479, -2.234128) (0.869542, -2.185691) (0.903747, -2.117381) (0.937505, -2.065369) (0.974026, -2.032184) (1.004619, -2.013355) (1.021479, -2.004765) knots 0 0 0 0 0 0 0.2 0.4 0.6 0.8 1 1 1 1 1 1
  spline S24 degree 5 poles (1.021479, -2.004765) (1.038338, -1.996174) (1.071553, -1.982492) (1.119867, -1.972451) (1.181788, -1.975712) (1.257157, -1.988191) (1.317541, -1.987487) (1.363676, -1.971824) (1.394932, -1.953086) (1.410685, -1.941641) knots -1 -1 -1 -1 -1 -1 -0.8 -0.6 -0.4 -0.2 0 0 0 0 0 0
  spline S25 degree 5 poles (1.410685, -1.941641) (1.426437, -1.930196) (1.453917, -1.90626) (1.483069, -1.867223) (1.502399, -1.810012) (1.513821, -1.734476) (1.529854, -1.674577) (1.554334, -1.631731) (1.577611, -1.60437) (1.59099, -1.59099) knots 0 0 0 0 0 0 0.2 0.4 0.6 0.8 1 1 1 1 1 1
  spline S26 degree 5 poles (1.59099, -1.59099) (1.60437, -1.577611) (1.631731, -1.554334) (1.674577, -1.529854) (1.734476, -1.513821) (1.810012, -1.502399) (1.867223, -1.483069) (1.90626, -1.453917) (1.930196, -1.426437) (1.941641, -1.410685) knots -1 -1 -1 -1 -1 -1 -0.8 -0.6 -0.4 -0.2 0 0 0 0 0 0
  spline S27 degree 5 poles (1.941641, -1.410685) (1.953086, -1.394932) (1.971824, -1.363676) (1.987487, -1.317541) (1.988191, -1.257157) (1.975712, -1.181788) (1.972451, -1.119867) (1.982492, -1.071553) (1.996174, -1.038338) (2.004765, -1.021479) knots 0 0 0 0 0 0 0.2 0.4 0.6 0.8 1 1 1 1 1 1
  spline S28 degree 5 poles (2.004765, -1.021479) (2.013355, -1.004619) (2.032184, -0.974026) (2.065369, -0.937505) (2.117381, -0.903747) (2.185691, -0.869542) (2.234128, -0.833479) (2.262246, -0.79369) (2.276519, -0.760159) (2.282536, -0.741641) knots -1 -1 -1 -1 -1 -1 -0.8 -0.6 -0.4 -0.2 0 0 0 0 0 0
  spline S29 degree 5 poles (2.282536, -0.741641) (2.288553, -0.723122) (2.296715, -0.687606) (2.297355, -0.638889) (2.279365, -0.581243) (2.244207, -0.513418) (2.22197, -0.455536) (2.21659, -0.406484) (2.219339, -0.370666) (2.222299, -0.351978) knots 0 0 0 0 0 0 0.2 0.4 0.6 0.8 1 1 1 1 1 1
  spline S30 degree 5 poles (2.222299, -0.351978) (2.225259, -0.333289) (2.233713, -0.298375) (2.253987, -0.253386) (2.293022, -0.205208) (2.347419, -0.151568) (2.382342, -0.102302) (2.396788, -0.055772) (2.4, -0.019472) (2.4, 0) knots -1 -1 -1 -1 -1 -1 -0.8 -0.6 -0.4 -0.2 0 0 0 0 0 0
  spline S31 degree 5 poles (2.4, 0) (2.4, 0.019472) (2.396788, 0.055772) (2.382342, 0.102302) (2.347419, 0.151568) (2.293022, 0.205208) (2.253987, 0.253386) (2.233713, 0.298375) (2.225259, 0.333289) (2.222299, 0.351978) knots 0 0 0 0 0 0 0.2 0.4 0.6 0.8 1 1 1 1 1 1
  spline S32 degree 5 poles (2.222299, 0.351978) (2.219339, 0.370666) (2.21659, 0.406484) (2.22197, 0.455536) (2.244207, 0.513418) (2.279365, 0.581243) (2.297355, 0.638889) (2.296715, 0.687606) (2.288553, 0.723122) (2.282536, 0.741641) knots -1 -1 -1 -1 -1 -1 -0.8 -0.6 -0.4 -0.2 0 0 0 0 0 0
  spline S33 degree 5 poles (2.282536, 0.741641) (2.276519, 0.760159) (2.262246, 0.79369) (2.234128, 0.833479) (2.185691, 0.869542) (2.117381, 0.903747) (2.065369, 0.937505) (2.032184, 0.974026) (2.013355, 1.004619) (2.004765, 1.021479) knots 0 0 0 0 0 0 0.2 0.4 0.6 0.8 1 1 1 1 1 1
  spline S34 degree 5 poles (2.004765, 1.021479) (1.996174, 1.038338) (1.982492, 1.071553) (1.972451, 1.119867) (1.975712, 1.181788) (1.988191, 1.257157) (1.987487, 1.317541) (1.971824, 1.363676) (1.953086, 1.394932) (1.941641, 1.410685) knots -1 -1 -1 -1 -1 -1 -0.8 -0.6 -0.4 -0.2 0 0 0 0 0 0
  spline S35 degree 5 poles (1.941641, 1.410685) (1.930196, 1.426437) (1.90626, 1.453917) (1.867223, 1.483069) (1.810012, 1.502399) (1.734476, 1.513821) (1.674577, 1.529854) (1.631731, 1.554334) (1.60437, 1.577611) (1.59099, 1.59099) knots 0 0 0 0 0 0 0.2 0.4 0.6 0.8 1 1 1 1 1 1
  spline S36 degree 5 poles (1.59099, 1.59099) (1.577611, 1.60437) (1.554334, 1.631731) (1.529854, 1.674577) (1.513821, 1.734476) (1.502399, 1.810012) (1.483069, 1.867223) (1.453917, 1.90626) (1.426437, 1.930196) (1.410685, 1.941641) knots -1 -1 -1 -1 -1 -1 -0.8 -0.6 -0.4 -0.2 0 0 0 0 0 0
  spline S37 degree 5 poles (1.410685, 1.941641) (1.394932, 1.953086) (1.363676, 1.971824) (1.317541, 1.987487) (1.257157, 1.988191) (1.181788, 1.975712) (1.119867, 1.972451) (1.071553, 1.982492) (1.038338, 1.996174) (1.021479, 2.004765) knots 0 0 0 0 0 0 0.2 0.4 0.6 0.8 1 1 1 1 1 1
  spline S38 degree 5 poles (1.021479, 2.004765) (1.004619, 2.013355) (0.974026, 2.032184) (0.937505, 2.065369) (0.903747, 2.117381) (0.869542, 2.185691) (0.833479, 2.234128) (0.79369, 2.262246) (0.760159, 2.276519) (0.741641, 2.282536) knots -1 -1 -1 -1 -1 -1 -0.8 -0.6 -0.4 -0.2 0 0 0 0 0 0
  spline S39 degree 5 poles (0.741641, 2.282536) (0.723122, 2.288553) (0.687606, 2.296715) (0.638889, 2.297355) (0.581243, 2.279365) (0.513418, 2.244207) (0.455536, 2.22197) (0.406484, 2.21659) (0.370666, 2.219339) (0.351978, 2.222299) knots 0 0 0 0 0 0 0.2 0.4 0.6 0.8 1 1 1 1 1 1
  circle A0 centre (0, 0) radius 1.25
  circle A1 centre (13.725, 0) radius 1
  line L0 (18.1, 9.5) -> (18.1, -9.5) construction
  circle A2 centre (0, 7.75) radius 1
  line L1 (15.784295, -2.493198) -> (0.269071, -3.640069)
  line L2 (4.4, 0.5) -> (3.615591, 0.5)
  circle A3 centre (0, 7.5) radius 2
  line L3 (18.1, -9.5) -> (-18.1, -9.5) construction
  circle A4 centre (-8.775, 0) radius 1
  line L4 (-15.784295, -2.493198) -> (-0.269071, -3.640069)
  circle A5 centre (0, 0) radius 3.65
  circle A6 centre (8.775, 0) radius 1
  line L5 (-15.784295, 2.493198) -> (-0.269071, 3.640069)
  circle A7 centre (6.3, 0) radius 1
  circle A8 centre (15.6, 0) radius 2.5
  line L6 (-4.4, 0) -> (-4.4, 0.5)
  line L7 (-4.4, -3.65) -> (4.4, -3.65) construction
  line L8 (-4.4, -2.334714) -> (-2.695836, -2.460685)
  line L9 (-4.4, 3.65) -> (-4.4, -3.65)
  circle A9 centre (0, 0) radius 1.25
  line L10 (0, 0) -> (-18.1, 0) construction
  line L11 (-4.4, -0.5) -> (-3.615591, -0.5)
  line L12 (-18.1, -9.5) -> (-18.1, 9.5) construction
  line L13 (-15.6, 0) -> (-16.2, 0) construction
  line L14 (-2, 7.5) -> (-2, -7.499995)
  circle A10 centre (-11.25, 0) radius 1
  line L15 (-4.4, 0.5) -> (-3.615591, 0.5)
  line L16 (0, 0) -> (0, 9.5) construction
  circle A11 centre (-16.2, 0) radius 1
  circle A12 centre (-15.6, 0) radius 2.5
  circle A13 centre (-6.3, 0) radius 1
  circle A14 centre (-13.725, 0) radius 1
  circle A15 centre (0, -5.25) radius 1
  circle A16 centre (0, -7.75) radius 1
  line L17 (-4.4, -3.65) -> (4.4, 3.65) construction
  line L18 (18.1, 9.5) -> (-18.1, -9.5) construction
  line L19 (-4.4, 2.334714) -> (-2.695836, 2.460685)
  circle A17 centre (0, 0) radius 2.325 construction
  line L20 (0, 7.5) -> (0, 7.75) construction
  line L21 (4.4, -3.65) -> (-4.4, 3.65) construction
  circle A18 centre (0, -7.5) radius 2
  line L22 (4.4, 3.334714) -> (4.4, 2.334714)
  line L23 (-18.1, 9.5) -> (18.1, -9.5) construction
  line L24 (4.4, -3.65) -> (4.4, 3.65)
  line L25 (4.4, -2.334714) -> (2.695836, -2.460685)
  line L26 (4.4, 3.65) -> (-4.4, 3.65) construction
  circle A19 centre (11.25, 0) radius 1
  line L27 (2, 7.5) -> (2, -7.499995)
  circle A20 centre (0, 5.25) radius 1
  line L28 (15.784295, 2.493198) -> (0.269071, 3.640069)
  line L29 (4.4, 2.334714) -> (2.695836, 2.460685)
  circle A21 centre (16.2, 0) radius 1
  line L30 (4.4, -0.5) -> (3.615591, -0.5)
  line L31 (-18.1, 9.5) -> (18.1, 9.5) construction
  line L32 (2, 7.5) -> (2, 3.053277)
  line L33 (-2, 7.5) -> (-2, 3.053277)
  line L34 (-2, -3.51212) -> (-2, -7.499995)
  line L35 (2, -7.499995) -> (2, -3.053277)
  dimension "d74" = 9.9
  dimension "d75" = 0
  dimension "d78" = 0
  dimension "d79" = -2.5
  dimension "OuterHubDia" = 7.3
  dimension "InnerHubDia" = 4.65
  dimension "MajorArmLen" = 36.2
  dimension "MinroArmLen" = 19
  dimension "TipDiaMajor" = 5
  dimension "TipDiaMinor" = 4
  dimension "ScrewHole" = 2.5
  dimension "DriveHole" = 2
  dimension "d14" = 2
  dimension "d19" = 8.8
  dimension "d90" = 7.3
  dimension "ReinforcerWidth" = 1
  dimension "d92" = 0.5
  dimension "HoleSlideAdj" = 0.6
  dimension "SideHoleSlideAdj" = 0.25
  constraint coincident A0.centre A5.centre
  constraint concentric A5 A17
  constraint horizontal L31
  constraint perpendicular L0 L31
  constraint parallel L3 L31
  constraint parallel L0 L12
  constraint coincident A0.centre L23
  constraint coincident A0.centre L18
  constraint midpoint L16.end L31
  constraint midpoint L10.end L12
  constraint coincident L10.end A12
  constraint coincident L13.start L10
  constraint coincident L16.end A3
  constraint coincident A3.centre L16
  constraint tangent L5 A12
  constraint tangent A5 L5
  constraint symmetric A3 L10 A18
  constraint coincident L14.start A3
  constraint vertical L14
  constraint tangent A3 L14
  constraint symmetric L14.start L27.start L16
  constraint symmetric A2 L10 A16
  constraint symmetric L10 A15 A20
  constraint symmetric A8 L16 A12
  constraint symmetric L16 A11 A21
  constraint symmetric A1 L16 A14
  constraint symmetric A10 L16 A19
  constraint symmetric A4 A6 L16
  constraint symmetric A7 L16 A13
  constraint horizontal L7
  constraint perpendicular L7 L24
  constraint parallel L7 L26
  constraint parallel L9 L24
  constraint coincident A0.centre L17
  constraint coincident A0.centre L21
  constraint parallel L22 L24
  constraint parallel L28 L29
  constraint midpoint L6.start L9
  constraint perpendicular L6 L10
  constraint perpendicular L6 L15
  constraint symmetric L6.end L11.start L10
  constraint symmetric L6.end L2.start L16
  constraint symmetric L11.start L30.start L16
  constraint coincident L13.start A12.centre
  constraint parallel L10 L13
  constraint coincident L13.end A11.centre
  constraint coincident A3.centre L20.start
  constraint parallel L16 L20
  constraint coincident A2.centre L20.end
  measures "OuterHubDia" diameter of A5
  measures "InnerHubDia" diameter of A17
  measures "MajorArmLen" distance of L0.end L3.end
  measures "MinroArmLen" distance of L0.start L0.end
  measures "TipDiaMajor" diameter of A12
  measures "TipDiaMinor" diameter of A3
  measures "ScrewHole" diameter of A9
  measures "DriveHole" diameter of A11
  measures "d14" diameter of A2
  measures "d19" distance of L17.end L9.start
  measures "d90" distance of L7.end L17.end
  measures "d92" distance of L6.start L6.end
  measures "HoleSlideAdj" distance of L13.end L13.start
  measures "SideHoleSlideAdj" distance of A3.centre A2.centre
extrude "Extrude1'" add sketch "Horn" against normal blind 2.7 separate body contours S0 S1 S2 S3 S4 S5 S6 S7 S34 S35 S36 S37 S38 S39 A5 L14 L27 | S27 S28 S29 S30 S31 S32 S33 S34 A5 L27 | S14 S15 S16 S17 S18 S19 S20 S21 S22 S23 S24 S25 S26 S27 A5 L14 L27 | S7 S8 S9 S10 S11 S12 S13 S14 A5 L14 picked at (-1.24671, 2.493427) picked at (2.756946, 0.413014) picked at (1.24671, -2.493427) picked at (-2.756946, -0.413014) makes body 9 in component "Horn"
extrude "Extrude2'" add sketch "Horn" along normal blind -1 and the other way blind -1.5 contours A5 L22 L24 L27 L28 L29 L32 | A5 L27 L28 L32 | L2 A5 L24 L29 | A3 A5 L5 L14 L27 A20 L28 L32 L33 | L1 A5 L27 L35 | L1 A5 L24 L25 L27 L35 | A5 L5 L14 L33 | A5 L5 L9 L14 L19 L33 | L2 A5 L24 L30 | A1 L1 A8 L22 L24 L28 | A3 A20 | L1 L4 A5 L14 A15 A18 L27 L34 L35 | A5 L24 L25 L30 | A5 L9 L15 L19 | L4 A5 L8 L9 L14 | L4 A5 L14 | A1 A8 | A15 A18 | A5 L6 L9 L11 L15 | L4 L5 L6 L9 A12 A14 | A5 L8 L9 L11 | A12 A14 picked at (3.831945, 2.710038) picked at (1.866237, 3.282217) picked at (4.109762, 1.255216) picked at (0.971744, 3.879663) picked at (1.866237, -3.282217) picked at (3.831945, -2.710038) picked at (-1.866237, 3.282217) picked at (-3.831945, 2.710038) picked at (4.15, 0) picked at (9.995155, -2.176879) picked at (0.859934, 6.343526) picked at (0.971744, -3.879663) picked at (4.109762, -1.255216) picked at (-4.109762, 1.255216) picked at (-3.831945, -2.710038) picked at (-1.866237, -3.282217) picked at (14.891208, 1.299154) picked at (0.859934, -6.343526) picked at (-4.148724, 0.222378) picked at (-9.995155, -2.176879) picked at (-4.109762, -1.255216) picked at (-14.891208, 1.299154) bodies 9 in component "Horn"
extrude "Extrude3''" add sketch "Horn" along normal blind 1.2 contours S0 S1 S2 S3 S4 S5 S6 S7 S14 S15 S16 S17 S18 S19 S20 S21 S22 S23 S24 S25 S26 S27 S34 S35 S36 S37 S38 S39 L14 L27 | S0 S1 S2 S3 S4 S5 S6 S7 S34 S35 S36 S37 S38 S39 A5 L14 L27 | S27 S28 S29 S30 S31 S32 S33 S34 A5 L27 | S27 S28 S29 S30 S31 S32 S33 S34 L27 | S14 S15 S16 S17 S18 S19 S20 S21 S22 S23 S24 S25 S26 S27 A5 L14 L27 | S7 S8 S9 S10 S11 S12 S13 S14 L14 | S7 S8 S9 S10 S11 S12 S13 S14 A5 L14 picked at (-1.75, 0) picked at (-1.24671, 2.493427) picked at (2.756946, 0.413014) picked at (2.077276, 0.117326) picked at (1.24671, -2.493427) picked at (-2.077276, -0.117326) picked at (-2.756946, -0.413014) bodies 9 in component "Horn"
extrude "Extrude4''" add sketch "Horn" along normal blind 2.3 contours S0 S1 S2 S3 S4 S5 S6 S7 S34 S35 S36 S37 S38 S39 A5 L14 L27 | S27 S28 S29 S30 S31 S32 S33 S34 A5 L27 | A5 L22 L24 L27 L28 L29 L32 | A5 L27 L28 L32 | S14 S15 S16 S17 S18 S19 S20 S21 S22 S23 S24 S25 S26 S27 A5 L14 L27 | S7 S8 S9 S10 S11 S12 S13 S14 A5 L14 | L1 A5 L27 L35 | L1 A5 L24 L25 L27 L35 | A5 L5 L14 L33 | A5 L5 L9 L14 L19 L33 | L2 A5 L24 L30 | L4 A5 L8 L9 L14 | L4 A5 L14 | A5 L6 L9 L11 L15 picked at (-1.24671, 2.493427) picked at (2.756946, 0.413014) picked at (3.831945, 2.710038) picked at (1.866237, 3.282217) picked at (1.24671, -2.493427) picked at (-2.756946, -0.413014) picked at (1.866237, -3.282217) picked at (3.831945, -2.710038) picked at (-1.866237, 3.282217) picked at (-3.831945, 2.710038) picked at (4.15, 0) picked at (-3.831945, -2.710038) picked at (-1.866237, -3.282217) picked at (-4.148724, 0.222378) bodies 9 in component "Horn"
chamfer "Chamfer1'" distance 0.766667 angle 45 6 edges at (4.4, 2.3, 0) (4.4, 2.3, -2.834714) (4.4, 2.3, 2.834714) (-4.4, 2.3, 2.834714) (-4.4, 2.3, 0) (-4.4, 2.3, -2.834714) on bodies 9 in component "Horn"
sketch "ServoOrigin" plane through (0, 0, 0) normal (0, 1, 0) x (-1, 0, 0) in component "Servo"
  circle A0 centre (0, 0) radius 1.25
sketch "Sketch1" plane through (0, 0, 0) normal (0, 1, 0) x (-1, 0, 0) in component "Joint"
  circle A0 centre (0, 0) radius 1.25